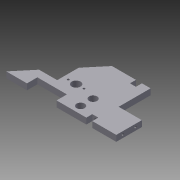
# Autodesk Inventor part: Inside Chassis3
Saved by Autodesk Inventor 2012 (Build 160160000, 160)
## iProperties
Created: 2012-04-02
Part Number: Inside Chassis3
Material: Aluminum-6061
Document SubType Name: Modeling
Designer: Jaime
Density: 2.71 g/cm^3
Mass: 223.634 g
Surface Area: 253.714 cm^2
Volume: 82.5218 cm^3
Author: Jaime
Autodesk Inventor part; units mm, degrees
ref_plane "YZ Plane" through (0, 0, 0) normal (1, 0, 0) x (0, 1, 0)
ref_plane "XZ Plane" through (0, 0, 0) normal (0, 1, 0) x (-1, 0, 0)
ref_plane "XY Plane" through (0, 0, 0) normal (0, 0, 1) x (1, 0, 0)
sketch "Sketch1" plane through (0, 0, 0) normal (0, 0, 1) x (1, 0, 0)
  line L0 (0, 0) -> (175, 0)
  line L1 (175, 0) -> (175, 91.44)
  line L2 (175, 91.44) -> (76.7273, 91.44)
  line L3 (76.7273, 91.44) -> (0, 0)
  dimension "d0" = 175
  dimension "d1" = 91.44
  dimension "d101" = 50
  constraints: 8 end point, 1 horizontal, 1 parallel, 1 perpendicular
  measures "d0" distance of L0.start L0.end
  measures "d1" distance of L0.end L1.end
  measures "d101" angle of L0 L3
extrude "Extrusion1" add sketch "Sketch1" along normal blind 9.525
sketch "Sketch11" plane through (0, 0, 0) normal (0, 0, -1) x (-1, 0, 0)
  circle A0 centre (-106.6758, 11.5887) radius 6.35 projected
  circle A1 centre (-106.6758, 11.5887) radius 6.9469 projected
  dimension "d121" = 12.7
  dimension "d122" = 13.8938
  measures "d121" diameter of A0
  measures "d122" diameter of A1
sketch "Sketch8" plane through (0, 0, 0) normal (0, 0, -1) x (-1, 0, 0)
  circle A0 centre (-73.1284, 38.046) radius 7 projected
  dimension "d105" = 14
  measures "d105" diameter of A0
sketch "Sketch9" plane through (0, 0, 0) normal (0, 0, -1) x (-1, 0, 0)
  circle A0 centre (-85.6284, 38.046) radius 1.25 projected
  circle A1 centre (-60.6284, 38.046) radius 1.25 projected
  constraints: 2 coincident
extrude "Extrusion2" cut sketch "Sketch8" against normal blind 9.525
hole "Hole7" at (85.6284, 38.046, 0) at (60.6284, 38.046, 0) direction (0, 0, 1) diameter 3.4036 end through all clearance for "Flat Head Machine Screw" size "M3" standard "Ansi Metric M Profile"
sketch "Sketch10" plane through (0, 0, 0) normal (0, 0, -1) x (-1, 0, 0)
  circle A0 centre (-106.6758, 31.4833) radius 6.35 projected
  dimension "d118" = 12.7
  measures "d118" diameter of A0
extrude "Extrusion3" cut sketch "Sketch10" against normal blind 9.525
extrude "Extrusion4" cut sketch "Sketch11" against normal blind 9.525 contours A0
sketch "Sketch12" plane through (0, 0, 0) normal (0, -1, 0) x (1, 0, 0)
  line L0 (175, 9.525) -> (0, 9.525) projected
  line L1 (0, 0) -> (175, 0) projected
  line L2 (33.02, 9.525) -> (80.01, 9.525)
  line L3 (80.01, 9.525) -> (80.01, 0)
  line L4 (80.01, 0) -> (33.02, 0)
  line L5 (33.02, 0) -> (33.02, 9.525)
  line L6 (175, 0) -> (175, 9.525) projected
  dimension "d126" = 46.99
  dimension "d196" = 94.99
  constraints: 8 end point, 2 parallel, 2 point on line, 1 horizontal, 1 perpendicular
  measures "d126" distance between parallel lines of L3 L5
  measures "d196" distance between parallel lines of L6 L3
extrude "Extrusion5" cut sketch "Sketch12" against normal blind 16.51 contours L3 L1 L5 L0
sketch "Sketch13" plane through (76.7273, 91.44, 0) normal (0, 1, 0) x (1, 0, 0)
  line L0 (98.2727, 0) -> (0, 0) projected
  line L1 (61.4427, 0) -> (98.2727, 0)
  line L2 (98.2727, 0) -> (98.2727, -9.525)
  line L3 (98.2727, -9.525) -> (61.4427, -9.525)
  line L4 (61.4427, -9.525) -> (61.4427, 0)
  point P0 (-76.7273, 0)
  dimension "d129" = 36.83
  constraints: 8 end point, 2 parallel, 1 horizontal, 1 perpendicular, 1 point on line
  measures "d129" distance between parallel lines of L2 L4
extrude "Extrusion6" cut sketch "Sketch13" against normal blind 50.8
sketch "Sketch14" plane through (76.7273, 91.44, 9.525) normal (0, 1, 0) x (1, 0, 0)
  line L0 (0, 9.525) -> (0, 0) projected
  line L1 (-76.7273, 0) -> (0, 0) projected
  line L2 (0, 9.525) -> (0, 0) projected
  line L3 (0, 9.525) -> (-76.7273, 9.525) projected
  line L4 (-76.7273, 9.525) -> (-76.7273, 0) projected
  line L5 (-24.13, 9.525) -> (-125.73, 9.525)
  line L6 (-125.73, 9.525) -> (-125.73, 0)
  line L7 (-125.73, 0) -> (-24.13, 0)
  line L8 (-24.13, 0) -> (-24.13, 9.525)
  dimension "d132" = 24.13
  dimension "d133" = 101.6
  constraints: 8 end point, 2 parallel, 2 point on line, 1 horizontal, 1 perpendicular
  measures "d132" distance between parallel lines of L0 L8
  measures "d133" distance between parallel lines of L8 L6
extrude "Extrusion7" cut sketch "Sketch14" against normal blind 62.992 contours L8 L1 L4 L3 | L4 L7 L6 L5
sketch "Sketch15" plane through (76.7273, 91.44, 9.525) normal (0, 1, 0) x (1, 0, 0)
  line L0 (61.4427, 9.525) -> (0, 9.525) projected
  line L1 (0, 9.525) -> (0, 0) projected
  line L2 (0, 0) -> (61.4427, 0) projected
  line L3 (38.1, 9.525) -> (47.625, 9.525)
  line L4 (47.625, 9.525) -> (47.625, 0)
  line L5 (47.625, 0) -> (38.1, 0)
  line L6 (38.1, 0) -> (38.1, 9.525)
  point P0 (-76.7273, 9.525)
  dimension "d136" = 9.525
  dimension "d137" = 38.1
  constraints: 8 end point, 2 parallel, 2 point on line, 1 horizontal, 1 perpendicular
  measures "d136" distance between parallel lines of L4 L6
  measures "d137" distance between parallel lines of L1 L6
extrude "Extrusion8" cut sketch "Sketch15" against normal blind 9.525 contours L4 L2 L6 L0
sketch "Sketch16" plane through (175, 0, 0) normal (0, -1, 0) x (1, 0, 0)
  line L0 (-94.99, 0) -> (0, 0) projected
  line L1 (0, 0) -> (0, 9.525) projected
  line L2 (0, 9.525) -> (-94.99, 9.525) projected
  line L3 (-47.625, 9.525) -> (-38.1, 9.525)
  line L4 (-38.1, 9.525) -> (-38.1, 0)
  line L5 (-38.1, 0) -> (-47.625, 0)
  line L6 (-47.625, 0) -> (-47.625, 9.525)
  point P0 (-175, 0)
  dimension "d140" = 38.1
  dimension "d141" = 9.525
  constraints: 8 end point, 2 parallel, 2 point on line, 1 horizontal, 1 perpendicular
  measures "d140" distance between parallel lines of L4 L1
  measures "d141" distance between parallel lines of L4 L6
extrude "Extrusion9" cut sketch "Sketch16" against normal blind 9.525 contours L6 L2 L4 L0
sketch "Sketch17" plane through (76.7273, 81.915, 9.525) normal (0, 1, 0) x (1, 0, 0)
  circle A0 centre (42.8625, 4.7625) radius 2.2479 projected
  point P0 (-76.7273, 9.525)
  constraints: 1 coincident
hole "Hole8" at (119.5898, 81.915, 4.7625) direction (0, -1, 0) diameter 3.302 depth 12.7 tip angle 118 thread size "8-32 UNC" class "2B" standard "ANSI Unified Screw Threads"
sketch "Sketch18" plane through (175, 9.525, 0) normal (0, -1, 0) x (1, 0, 0)
  circle A0 centre (-42.8625, 4.7625) radius 2.2479 projected
  point P0 (-175, 0)
  constraints: 1 coincident
hole "Hole9" at (132.1375, 9.525, 4.7625) direction (0, 1, 0) diameter 3.302 depth 12.7 tip angle 118 thread size "8-32 UNC" class "2B" standard "ANSI Unified Screw Threads"
sketch "Sketch19" plane through (76.7273, 40.64, 0) normal (0, 1, 0) x (1, 0, 0)
  circle A0 centre (71.6027, -4.7625) radius 2.2479 projected
  circle A1 centre (89.3827, -4.7625) radius 2.2479 projected
  point P0 (-76.7273, 0)
  constraints: 2 coincident
hole "Hole10" at (148.33, 40.64, 4.7625) at (166.11, 40.64, 4.7625) direction (0, -1, 0) diameter 3.302 depth 12.7 tip angle 118 thread size "8-32 UNC" class "2B" standard "ANSI Unified Screw Threads"
sketch "Sketch20" plane through (175, 0, 9.525) normal (1, 0, 0) x (0, 0, -1)
  line L0 (9.525, 40.64) -> (0, 40.64) projected
  line L1 (9.525, 0) -> (0, 0) projected
  point P0 (4.7625, 10.16)
  point P1 (4.7625, 30.48)
  dimension "d165" = 30.48
  dimension "d166" = 10.16
  dimension "d167" = 10.16
  measures "d165" distance from line of L1 point (4.763, 30.48)
  measures "d166" distance from line of L1 point (4.763, 10.16)
  measures "d167" distance from line of point (4.763, 30.48) L0
hole "Hole11" at (175, 10.16, 4.7625) at (175, 30.48, 4.7625) direction (-1, 0, 0) diameter 3.302 depth 12.7 tip angle 118 thread size "8-32 UNC" class "2B" standard "ANSI Unified Screw Threads"
sketch "Sketch21" plane through (52.5973, 28.448, 0) normal (-1, 0, 0) x (0, 0, 1)
  circle A0 centre (3.79, 4.06) radius 1.0795 projected
  circle A1 centre (3.79, 4.06) radius 1.55 projected
  circle A2 centre (44.49, 20.36) radius 1.55 projected
  line L0 (46.99, 22.86) -> (46.99, 1.56) projected
  line L1 (1.29, 22.86) -> (46.99, 22.86) projected
  line L2 (1.29, 1.56) -> (1.29, 22.86) projected
  line L3 (46.99, 1.56) -> (1.29, 1.56) projected
  line L4 (1.29, 12.21) -> (46.99, 12.21)
  circle A3 centre (3.79, 20.36) radius 1.0795
  point P0 (0, -28.448)
  constraints: 2 coincident, 2 end point, 2 midpoint, 1 centre point
hole "Hole12" at (52.5973, 48.808, 3.79) at (52.5973, 32.508, 3.79) direction (1, 0, 0) diameter 2.159 depth 5.08 tip angle 118
sketch "Sketch22" plane through (76.7273, 91.44, 0) normal (-0.7660444, 0.6427876, 0) x (0, 0, 1)
  circle A0 centre (4.7625, -7.62) radius 2.159 projected
  circle A1 centre (4.7625, -33.02) radius 2.159 projected
  circle A2 centre (4.7625, -84.7725) radius 2.2479 projected
  point P0 (0, -119.3664)
  constraints: 3 coincident
hole "Hole13" at (71.8292, 85.6027, 4.7625) at (55.5024, 66.1452, 4.7625) at (22.2366, 26.5005, 4.7625) direction (0.7660444, -0.6427876, 0) diameter 3.302 depth 5.08 tip angle 118 thread size "8-32 UNC" class "2B" standard "ANSI Unified Screw Threads"
sketch "Sketch23" plane through (0, 0, 0) normal (-0.7660444, 0.6427876, 0) x (0, 0, 1)
  circle A0 centre (4.7625, 24.1164) radius 2.159 projected
  constraints: 1 coincident
hole "Hole14" at (15.5018, 18.4743, 4.7625) direction (0.7660444, -0.6427876, 0) diameter 3.302 depth 7.62 tip angle 118 thread size "8-32 UNC" class "2B" standard "ANSI Unified Screw Threads"
body "Solid1"
